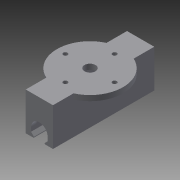
# Autodesk Inventor part: CarFrontAxel
Saved by Autodesk Inventor 2015 (Build 190159000, 159)
## iProperties
Created: 2016-04-06
Part Number: CarFrontAxel
Material: Generic
Document SubType Name: Modeling
Designer: Lee
Density: 1 g/cm^3
Appearance: Default
Author: Lee
Autodesk Inventor part; units mm, degrees
ref_plane "YZ Plane" through (0, 0, 0) normal (1, 0, 0) x (0, 1, 0)
ref_plane "XZ Plane" through (0, 0, 0) normal (0, 1, 0) x (-1, 0, 0)
ref_plane "XY Plane" through (0, 0, 0) normal (0, 0, 1) x (1, 0, 0)
sketch "Sketch1" plane through (0, 0, 0) normal (0, 0, 1) x (1, 0, 0)
  line L0 (0, 0) -> (8.2, 0)
  line L1 (8.2, 0) -> (8.2, 30.48)
  line L2 (8.2, 30.48) -> (0, 30.48)
  line L3 (0, 30.48) -> (0, 0)
  line L4 (6.6, 28.88) -> (6.6, 1.6)
  line L5 (6.6, 1.6) -> (1.6, 1.6)
  line L6 (1.6, 1.6) -> (1.6, 28.88)
  line L7 (1.6, 28.88) -> (6.6, 28.88)
  dimension "d0" = 30.48
  dimension "d1" = 8.2
  dimension "d2" = 1.6
  constraints: 16 end point, 4 parallel, 2 perpendicular, 1 horizontal, 3 other
  measures "d0" distance of L0.end L1.end
  measures "d1" distance of L0.start L0.end
  measures "d2" distance between parallel lines of L1 L4
extrude "Extrusion1" add sketch "Sketch1" along normal blind 11.4
sketch "Sketch2" plane through (0, 0, 0) normal (0, -1, 0) x (1, 0, 0)
  line L0 (6.6, 0) -> (6.6, 11.4) projected
  line L1 (1.6, 0) -> (1.6, 11.4) projected
  line L2 (0, 0) -> (8.2, 0) projected
  line L3 (1.6, 0) -> (1.6, 2.4)
  line L4 (1.6, 0) -> (1.6, 11.4) projected
  line L5 (6.6, 0) -> (6.6, 2.4)
  line L6 (6.6, 0) -> (6.6, 11.4) projected
  line L7 (1.6, 0) -> (6.6, 0)
  arc A0 (6.6, 2.4) -> (1.6, 2.4) centre (4.1, 2.4) ccw
  dimension "d5" = 2.4
  dimension "d6" = 2.4
  constraints: 6 end point, 2 point on circle, 2 point on line, 1 centre point, 1 tangent
  measures "d5" distance of L1.start L3.end
  measures "d6" distance of L0.start L5.end
extrude "Extrusion2" cut sketch "Sketch2" against normal up to surface (30.48 mm away)
sketch "Sketch3" plane through (0, 0, 0) normal (-1, 0, 0) x (0, 0, 1)
  line L0 (0, 30.48) -> (0, 0) projected
  line L1 (0, 0) -> (11.4, 0) projected
  line L2 (11.4, 30.48) -> (11.4, 0) projected
  line L3 (0, 30.48) -> (11.4, 30.48) projected
  line L4 (0, 0) -> (11.4, 0) projected
  line L5 (11.4, 30.48) -> (9.8, 30.48)
  line L6 (9.8, 30.48) -> (9.8, 0)
  line L7 (9.8, 0) -> (11.4, 0)
  line L8 (11.4, 0) -> (11.4, 30.48)
  dimension "d9" = 1.6
  constraints: 8 end point, 2 parallel, 1 horizontal, 1 perpendicular, 1 point on line
  measures "d9" distance of L7.end L6.end
extrude "Extrusion3" add sketch "Sketch3" against normal up to next contours L3 L2 L1 L6
sketch "Sketch4" plane through (0, 0, 11.4) normal (0, 0, 1) x (1, 0, 0)
  line L0 (0, 0) -> (8.2, 0) projected
  line L1 (8.2, 0) -> (8.2, 30.48) projected
  line L2 (8.2, 30.48) -> (0, 30.48) projected
  line L3 (0, 30.48) -> (0, 0) projected
  line L4 (6.6, 0) -> (1.6, 0) projected
  line L5 (4.1, 0) -> (4.1, 30.48)
  line L6 (1.6, 30.48) -> (6.6, 30.48) projected
  line L7 (8.2, 0) -> (0, 30.48)
  line L8 (8.2, 30.48) -> (0, 0) construction
  circle A0 centre (4.1, 7.84) radius 0.65
  circle A1 centre (4.1, 22.64) radius 0.65
  point P0 (4.1, 15.24)
  dimension "d12" = 7.4
  dimension "d13" = 7.4
  dimension "d14" = 1.3
  dimension "d15" = 1.3
  constraints: 6 end point, 3 midpoint, 2 centre point, 2 point on line
  measures "d12" distance of point (4.1, 15.24) A0.centre
  measures "d13" distance of point (4.1, 15.24) A1.centre
  measures "d14" diameter of A0
  measures "d15" diameter of A1
extrude "Extrusion4" cut sketch "Sketch4" against normal up to next contours A0 L5 | L5 A0 | A1 L5 | L5 A1
sketch "Sketch5" plane through (0, 0, 11.4) normal (0, 0, 1) x (1, 0, 0)
  circle A0 centre (4.1, 7.84) radius 0.65 projected
  circle A1 centre (4.1, 22.64) radius 0.65 projected
  line L0 (0, 0) -> (8.2, 0) projected
  line L1 (8.2, 0) -> (8.2, 30.48) projected
  line L2 (8.2, 30.48) -> (0, 30.48) projected
  line L3 (0, 30.48) -> (0, 0) projected
  line L4 (8.2, 0) -> (0, 30.48)
  line L5 (0, 0) -> (8.2, 30.48)
  circle A2 centre (4.1, 15.24) radius 9.935
  dimension "d18" = 19.87
  constraints: 4 end point, 1 centre point, 1 coincident, 1 midpoint
  measures "d18" diameter of A2
extrude "Extrusion5" add sketch "Sketch5" against normal blind 1.6 contours A2 L3 | L3 A2 L4 L5 | L5 L4 A2 | A2 L4 L5 L1 | L1 A2 | L4 A2 L5
sketch "Sketch6" plane through (0, 0, 11.4) normal (0, 0, 1) x (1, 0, 0)
  line L0 (1.6, 28.88) -> (1.6, 1.6) projected
  circle A0 centre (4.1, 22.64) radius 0.65 projected
  circle A1 centre (4.1, 7.84) radius 0.65 projected
  line L1 (0, 6.1905) -> (0, 0) projected
  line L2 (0, 0) -> (8.2, 0) projected
  line L3 (8.2, 0) -> (8.2, 6.1905) projected
  arc A2 (8.2, 6.1905) -> (8.2, 24.2895) centre (4.1, 15.24) ccw projected
  line L4 (8.2, 24.2895) -> (8.2, 30.48) projected
  line L5 (8.2, 30.48) -> (0, 30.48) projected
  line L6 (0, 30.48) -> (0, 24.2895) projected
  arc A3 (0, 24.2895) -> (0, 6.1905) centre (4.1, 15.24) ccw projected
  line L7 (8.2, 0) -> (0, 30.48)
  line L8 (8.2, 30.48) -> (0, 0)
  arc A4 (0, 24.2895) -> (0, 6.1905) centre (4.1, 15.24) ccw projected
  line L9 (-5.835, 15.24) -> (14.035, 15.24) construction
  arc A5 (8.2, 6.1905) -> (8.2, 24.2895) centre (4.1, 15.24) ccw projected
  circle A6 centre (-3.3, 15.24) radius 0.65
  circle A7 centre (11.5, 15.24) radius 0.65
  dimension "d21" = 7.4
  dimension "d22" = 7.4
  dimension "d23" = 1.3
  dimension "d24" = 1.3
  constraints: 6 end point, 4 point on circle, 2 centre point, 2 point on line
  measures "d21" distance of A2.centre A6.centre
  measures "d22" distance of A2.centre A7.centre
  measures "d23" diameter of A6
  measures "d24" diameter of A7
extrude "Extrusion6" cut sketch "Sketch6" against normal up to next contours A6 | A7
sketch "Sketch7" plane through (0, 0, 11.4) normal (0, 0, 1) x (1, 0, 0)
  circle A0 centre (11.5, 15.24) radius 0.65 projected
  circle A1 centre (-3.3, 15.24) radius 0.65 projected
  circle A2 centre (4.1, 22.64) radius 0.65 projected
  circle A3 centre (4.1, 7.84) radius 0.65 projected
  line L0 (0, 6.1905) -> (0, 0) projected
  line L1 (0, 0) -> (8.2, 0) projected
  line L2 (8.2, 0) -> (8.2, 6.1905) projected
  arc A4 (8.2, 6.1905) -> (8.2, 24.2895) centre (4.1, 15.24) ccw projected
  line L3 (8.2, 24.2895) -> (8.2, 30.48) projected
  line L4 (8.2, 30.48) -> (0, 30.48) projected
  line L5 (0, 30.48) -> (0, 24.2895) projected
  arc A5 (0, 24.2895) -> (0, 6.1905) centre (4.1, 15.24) ccw projected
  line L6 (0, 0) -> (8.2, 30.48)
  line L7 (0, 30.48) -> (8.2, 0)
  circle A6 centre (4.1, 15.24) radius 1.65
  dimension "d27" = 3.3
  constraints: 4 end point, 1 centre point, 1 coincident
  measures "d27" diameter of A6
extrude "Extrusion7" cut sketch "Sketch7" against normal blind 1.6 contours A6 L7 L6 | L6 L7 A6 | L7 L6 A6 | L7 A6 L6
sketch "Sketch8" plane through (6.6, 30.48, 0) normal (0, 1, 0) x (1, 0, 0)
  line L0 (-5, -2.4) -> (-5, 0) projected
  line L1 (0, 0) -> (0, -2.4) projected
  line L2 (-5, -1.2) -> (-3.8, 0)
  line L3 (-5, -1.2) -> (-2.8401, -1.2) construction
  line L4 (-5, 0) -> (-3.8, 0)
  line L5 (0, -1.2) -> (-1.2, 0)
  line L6 (0, 0) -> (-1.2, 0)
  point P0 (-6.6, 0)
  dimension "d30" = 45
  constraints: 10 end point, 2 midpoint, 1 horizontal
  measures "d30" angle of L3 L2
extrude "Extrusion8" add sketch "Sketch8" against normal up to surface (30.48 mm away)
fillet "Fillet1" radius 0.2 2 edges at (2.8, 15.24, 0) (5.4, 15.24, 0)
body "Solid1"
